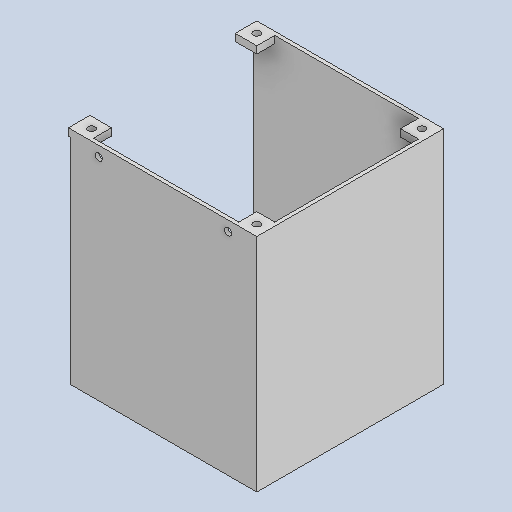
# Autodesk Inventor part: Low
Saved by Autodesk Inventor 2025 (Build 290162000, 162)
## iProperties
Created: 2025-08-07
Part Number: Low
Material: Generic
Document SubType Name: Modeling
Designer: Pravoslav
Density: 1 g/cm^3
Appearance: Default
Author: Pravoslav
Autodesk Inventor part; units mm, degrees
ref_plane "YZ Plane" through (0, 0, 0) normal (1, 0, 0) x (0, 1, 0)
ref_plane "XZ Plane" through (0, 0, 0) normal (0, 1, 0) x (-1, 0, 0)
ref_plane "XY Plane" through (0, 0, 0) normal (0, 0, 1) x (1, 0, 0)
sketch "Sketch1" plane through (0, 0, 0) normal (0, 1, 0) x (-1, 0, 0)
  line L0 (65, 65) -> (-65, 65)
  line L1 (-65, 65) -> (-65, -65)
  line L2 (-65, -65) -> (65, -65)
  line L3 (65, -65) -> (65, 65)
  line L4 (65, 65) -> (-65, -65) construction
  line L5 (-65, 65) -> (65, -65) construction
  line L6 (55.5, 55.5) -> (-55.5, 55.5)
  line L7 (-55.5, 55.5) -> (-55.5, -55.5)
  line L8 (-55.5, -55.5) -> (55.5, -55.5)
  line L9 (55.5, -55.5) -> (55.5, 55.5)
  line L10 (55.5, 55.5) -> (-55.5, -55.5) construction
  line L11 (-55.5, 55.5) -> (55.5, -55.5) construction
  circle A0 centre (55.5, 55.5) radius 2.5
  circle A1 centre (55.5, -55.5) radius 2.5
  circle A2 centre (-55.5, -55.5) radius 2.5
  circle A3 centre (-55.5, 55.5) radius 2.5
  point P0 (0, 0)
  dimension "d0" = 130
  dimension "d1" = 130
  dimension "d2" = 111
  dimension "d3" = 5
  dimension "d4" = 5
  dimension "d5" = 5
  dimension "d6" = 5
  constraints: 24 end point, 4 centre point, 4 midpoint, 4 parallel, 3 coincident, 2 horizontal, 2 perpendicular, 2 point on line
  measures "d0" distance of L2.end L1.end
  measures "d1" distance of L1.end L0.end
  measures "d2" distance of L8.end L7.end
  measures "d3" diameter of A0
  measures "d4" diameter of A1
  measures "d5" diameter of A2
  measures "d6" diameter of A3
extrude "Extrusion1" add sketch "Sketch1" along normal blind 4 contours L3 L2 L1 L0 | L6 A0 L9 A1 L8 A2 L7 A3
sketch "Sketch2" plane through (0, 4, 0) normal (0, 1, 0) x (1, 0, 0)
  line L0 (-62.5, -62.5) -> (62.5, -62.5)
  line L1 (62.5, -62.5) -> (62.5, 62.5)
  line L2 (62.5, 62.5) -> (-62.5, 62.5)
  line L3 (-62.5, 62.5) -> (-62.5, -62.5)
  line L4 (-62.5, -62.5) -> (62.5, 62.5) construction
  line L5 (62.5, -62.5) -> (-62.5, 62.5) construction
  line L6 (65, -65) -> (65, 65) projected
  line L7 (-65, -65) -> (65, -65)
  line L8 (65, -65) -> (65, 65)
  line L9 (65, 65) -> (-65, 65)
  line L10 (-65, 65) -> (-65, -65)
  line L11 (-65, -65) -> (65, 65) construction
  line L12 (65, -65) -> (-65, 65) construction
  line L13 (-62.5, -62.5) -> (-65, -62.5)
  line L14 (-62.5, 62.5) -> (-65, 62.5)
  point P0 (0, 0)
  dimension "d9" = 125
  dimension "d10" = 125
  constraints: 28 end point, 4 midpoint, 4 parallel, 4 perpendicular, 2 horizontal, 2 point on line
  measures "d9" distance of L2.end L1.end
  measures "d10" distance of L1.end L0.end
extrude "Extrusion2" add sketch "Sketch2" along normal blind 150 contours L0 L1 L2 L14 L10 L9 L6 L7 L13
sketch "Sketch3" plane through (-65, 0, 65) normal (0, 0, 1) x (1, 0, 0)
  circle A0 centre (20, 147) radius 2.5
  circle A1 centre (110, 147) radius 2.5
  line L0 (0, 154) -> (130, 154) projected
  line L1 (130, 0) -> (130, 154) projected
  line L2 (0, 0) -> (0, 154) projected
  point P0 (65, 0)
  dimension "d13" = 5
  dimension "d14" = 5
  dimension "d15" = 7
  dimension "d16" = 7
  dimension "d17" = 20
  dimension "d18" = 20
  constraints: 2 centre point
  measures "d13" diameter of A0
  measures "d14" diameter of A1
  measures "d15" distance from line of L0 A0.centre
  measures "d16" distance from line of L0 A1.centre
  measures "d17" distance from line of L1 A1.centre
  measures "d18" distance from line of L2 A0.centre
extrude "Extrusion3" cut sketch "Sketch3" against normal up to surface (2.5 mm away)
sketch "Sketch4" plane through (-65, 0, -65) normal (-1, 0, 0) x (0, 0, 1)
  line L0 (130, 0) -> (130, 154) projected
  line L1 (130, 109) -> (116, 109)
  line L2 (116, 109) -> (116, 69)
  line L3 (116, 69) -> (130, 69)
  line L4 (130, 69) -> (130, 109)
  circle A0 centre (122, 99.5) radius 2.5
  circle A1 centre (122, 78.5) radius 2.5
  line L5 (2.5, 154) -> (127.5, 154) projected
  point P0 (65, 0)
  point P1 (123, 109)
  dimension "d21" = 14
  dimension "d22" = 40
  dimension "d23" = 5
  dimension "d24" = 5
  dimension "d25" = 21
  dimension "d27" = 6
  dimension "d28" = 9.5
  dimension "d29" = 45
  constraints: 8 end point, 2 centre point, 2 parallel, 1 horizontal, 1 midpoint, 1 perpendicular, 1 point on line
  measures "d21" distance of L3.end L2.end
  measures "d22" distance of L2.end L1.end
  measures "d23" diameter of A0
  measures "d24" diameter of A1
  measures "d25" distance of A1.centre A0.centre
  measures "d27" distance from line of L2 A0.centre
  measures "d28" distance from line of L1 A0.centre
  measures "d29" distance between parallel lines of L5 L1
extrude "Extrusion4" add sketch "Sketch4" against normal blind 5
sketch "Sketch5" plane through (0, 154, 0) normal (0, 1, 0) x (1, 0, 0)
  line L0 (65, -65) -> (65, 65) projected
  line L1 (65, 65) -> (50, 65)
  line L2 (50, 65) -> (50, 50)
  line L3 (50, 50) -> (65, 50)
  line L4 (65, 50) -> (65, 65)
  line L5 (65, -65) -> (50, -65)
  line L6 (50, -65) -> (50, -50)
  line L7 (50, -50) -> (65, -50)
  line L8 (65, -50) -> (65, -65)
  line L9 (-66.1147, -65) -> (-51.1147, -65)
  line L10 (-51.1147, -65) -> (-51.1147, -50)
  line L11 (-51.1147, -50) -> (-66.1147, -50)
  line L12 (-66.1147, -50) -> (-66.1147, -65)
  line L13 (-65, 65) -> (-50, 65)
  line L14 (-50, 65) -> (-50, 50)
  line L15 (-50, 50) -> (-65, 50)
  line L16 (-65, 50) -> (-65, 65)
  line L17 (57.5, 57.5) -> (-57.5, 57.5)
  line L18 (-57.5, 57.5) -> (-57.5, -57.5)
  line L19 (-57.5, -57.5) -> (57.5, -57.5)
  line L20 (57.5, -57.5) -> (57.5, 57.5)
  line L21 (57.5, 57.5) -> (-57.5, -57.5) construction
  line L22 (-57.5, 57.5) -> (57.5, -57.5) construction
  circle A0 centre (57.5, 57.5) radius 2.5
  circle A1 centre (57.5, -57.5) radius 2.5
  circle A2 centre (-57.5, -57.5) radius 2.5
  circle A3 centre (-57.5, 57.5) radius 2.5
  point P0 (0, 0)
  point P1 (0, -57.5)
  dimension "d32" = 15
  dimension "d33" = 15
  dimension "d34" = 15
  dimension "d35" = 15
  dimension "d36" = 15
  dimension "d37" = 15
  dimension "d38" = 15
  dimension "d39" = 15
  dimension "d40" = 5
  dimension "d41" = 5
  dimension "d42" = 5
  dimension "d43" = 5
  dimension "d46" = 115
  dimension "d47" = 115
  constraints: 44 end point, 10 parallel, 5 horizontal, 5 perpendicular, 4 centre point, 4 coincident, 3 midpoint, 2 point on line
  measures "d32" distance of L3.end L2.end
  measures "d33" distance of L2.end L1.end
  measures "d34" distance of L6.end L7.end
  measures "d35" distance of L5.end L6.end
  measures "d36" distance of L11.end L10.end
  measures "d37" distance of L10.end L9.end
  measures "d38" distance of L14.end L15.end
  measures "d39" distance of L13.end L14.end
  measures "d40" diameter of A0
  measures "d41" diameter of A1
  measures "d42" diameter of A2
  measures "d43" diameter of A3
  measures "d46" distance from line of point (0, -57.5) L17
  measures "d47" distance between parallel lines of L18 L20
extrude "Extrusion5" add sketch "Sketch5" against normal blind 5 contours L5 L6 L19 A1 L20 L7 L0 | L3 L20 A0 L17 L2 L1 L0 | L20 A1 L19 L6 L7 | L3 L2 L17 A0 L20 | L19 A2 L18 L11 L10 | L10 L9 L12 L11 L18 A2 L19 | L17 A3 L18 L15 L16 L13 L14 | L14 L15 L18 A3 L17
body "Solid1"
